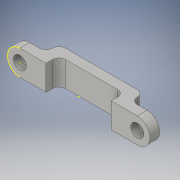
# Autodesk Inventor part: opencm_strap
Saved by Autodesk Inventor 2016 (Build 200138000, 138)
## iProperties
Created: 2016-02-15
Part Number: opencm_strap
Material: Generic
Document SubType Name: Modeling
Designer: jforce
Density: 1 g/cm^3
Appearance: Default
Author: jforce
Autodesk Inventor part; units mm, degrees
ref_plane "YZ Plane" through (0, 0, 0) normal (1, 0, 0) x (0, 1, 0)
ref_plane "XZ Plane" through (0, 0, 0) normal (0, 1, 0) x (-1, 0, 0)
ref_plane "XY Plane" through (0, 0, 0) normal (0, 0, 1) x (1, 0, 0)
sketch "Sketch1" plane through (0, 0, 0) normal (0, 0, 1) x (1, 0, 0)
  line L0 (-18, 0) -> (18, 0) construction
  arc A0 (-18, 3.8571) -> (-18, -3.8571) centre (-18, 0) ccw
  arc A1 (18, -3.8571) -> (18, 3.8571) centre (18, 0) ccw
  line L1 (-18, -3.8571) -> (18, -3.8571)
  line L2 (18, 3.8571) -> (-18, 3.8571)
  point P0 (0, 0)
  dimension "d26" = 36
  constraints: 6 end point, 4 point on circle, 2 centre point, 2 coincident, 2 horizontal, 1 parallel
  measures "d26" distance of A1.centre A0.centre
extrude "Extrusion1" add sketch "Sketch1" along normal blind 7
sketch "Sketch2" plane through (-18, 3.8571, 0) normal (0, 1, 0) x (1, 0, 0)
  line L0 (33, -4) -> (50.7344, -4) construction
  line L1 (36, -7) -> (0, -7) projected
  line L2 (10, -3) -> (26, -3)
  line L3 (28, -5) -> (28, -7)
  line L4 (28, -7) -> (8, -7)
  line L5 (8, -7) -> (8, -5)
  line L6 (36, 0) -> (0, 0) projected
  line L7 (0, 0) -> (0, -7) projected
  line L8 (36, 0) -> (36, -7) projected
  line L9 (3, -4) -> (-4.7246, -4)
  line L10 (-4.7246, -4) -> (-4.7246, 3)
  line L11 (-4.7246, 3) -> (5, 3)
  line L12 (5, 3) -> (5, -2)
  line L13 (33, -4) -> (47.7116, -4)
  line L14 (47.7116, -4) -> (47.7116, 0.5212)
  line L15 (47.7116, 0.5212) -> (31, 0.5212)
  line L16 (31, 0.5212) -> (31, -2)
  arc A0 (3, -4) -> (5, -2) centre (3, -2) ccw
  arc A1 (10, -3) -> (8, -5) centre (10, -5) ccw
  arc A2 (28, -5) -> (26, -3) centre (26, -5) ccw
  arc A3 (31, -2) -> (33, -4) centre (33, -2) ccw
  point P0 (18, 0)
  point P1 (8, -3)
  point P2 (28, -3)
  point P3 (5, -4)
  dimension "d7" = 3
  dimension "d8" = 8
  dimension "d9" = 8
  dimension "d10" = 3
  dimension "d11" = 3
  dimension "d24" = 2
  constraints: 26 end point, 8 point on circle, 8 point on line, 8 tangent, 6 parallel, 4 centre point, 4 horizontal, 3 equal radius, 3 perpendicular
  measures "d7" distance between parallel lines of L6 L2
  measures "d8" distance between parallel lines of L7 L5
  measures "d9" distance between parallel lines of L3 L8
  measures "d10" distance between parallel lines of L12 L5
  measures "d11" distance between parallel lines of L16 L3
  measures "d24" radius of A0
extrude "Extrusion2" cut sketch "Sketch2" against normal blind 10 contours L1 L5 A1 L2 A2 L3 | L13 A3 L16 L6 L8 | L8 L6 L16 L15 L14 L13 | L9 L10 L11 L12 L6 L7 | L7 L6 L12 A0 L9
sketch "Sketch3" plane through (0, 0, 7) normal (0, 0, 1) x (1, 0, 0)
  arc A0 (-18, 3.8571) -> (-18, -3.8571) centre (-18, 0) ccw projected
  point P0 (0, 0)
sketch "Sketch4" plane through (-13, 3.8571, 4) normal (0, 0, -1) x (-1, 0, 0)
  arc A0 (5, -7.7143) -> (5, 0) centre (5, -3.8571) ccw projected
  point P0 (-13, -3.8571)
hole "Hole1" at (-18, 0, 4) direction (0, 0, 1) diameter 4 depth 3 tip angle 118 counterbore diameter 5 counterbore depth 0.85
pattern_linear "Rectangular Pattern1" count 2 spacing 36 along (1, 0, 0) of "Hole1"
fillet "Fillet1" radius 2 2 edges at (13, 0, 0) (-13, 0, 0)
body "Solid1"
